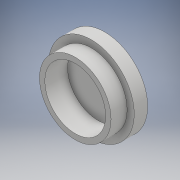
# Autodesk Inventor part: CapForPh
Saved by Autodesk Inventor 2019 (Build 230136000, 136)
## iProperties
Created: 2017-07-24
Part Number: CapForPh
Material: Generic
Document SubType Name: Modeling
Designer: steele
Density: 1 g/cm^3
Appearance: Default
Author: steele
Autodesk Inventor part; units mm, degrees
ref_plane "YZ Plane" through (0, 0, 0) normal (1, 0, 0) x (0, 1, 0)
ref_plane "XZ Plane" through (0, 0, 0) normal (0, 1, 0) x (-1, 0, 0)
ref_plane "XY Plane" through (0, 0, 0) normal (0, 0, 1) x (1, 0, 0)
sketch "Sketch2" plane through (0, 0, 0) normal (0, 0, 1) x (1, 0, 0)
  line L0 (0, 0) -> (0, 11) construction
  line L1 (0, 11) -> (-16, 11)
  line L2 (-16, 11) -> (-16, 6)
  line L3 (-16, 6) -> (-13.35, 6)
  line L4 (-13.35, 6) -> (-13.35, 0)
  line L5 (-13.35, 0) -> (-11.35, 0)
  line L6 (0, 0) -> (-13.35, 0) construction
  line L7 (-11.35, 0) -> (-11.35, 6)
  line L8 (0, 11) -> (0, 8.5)
  line L9 (-11.35, 8.5) -> (-11.35, 6)
  line L10 (-11.35, 8.5) -> (0, 8.5)
  dimension "d4" = 16
  dimension "d5" = 5
  dimension "d6" = 6
  dimension "d8" = 13.35
  dimension "d16" = 11.35
  dimension "d17" = 2
  constraints: 22 end point, 5 perpendicular, 3 vertical, 2 point on line, 1 collinear, 1 horizontal, 1 parallel
  measures "d4" distance of L0.end L1.end
  measures "d5" distance of L1.end L2.end
  measures "d6" distance of L3.end L4.end
  measures "d8" distance between parallel lines of L0 L4
  measures "d16" distance between parallel lines of L7 L0
  measures "d17" distance between parallel lines of L7 L4
revolve "Revolution1" add sketch "Sketch2" angle 360 about axis through (0, 0, 0) along (0, 1, 0)
sketch "Sketch4" plane through (0, 11, 0) normal (0, 1, 0) x (1, 0, 0)
  circle A0 centre (0, 0) radius 16 construction
  line L0 (-16, 0) -> (16, 0) construction
  spline S0 degree 2 poles (-9.9681, -0.6371) (-9.9681, -1.7395) (-11.0853, -3.089) (-11.9059, -3.089) knots 0 0 0 1 2 2 2
  spline S1 degree 2 poles (-11.9059, -3.089) (-12.247, -3.089) (-12.7561, -2.9357) (-13.0428, -2.7677) knots 0 0 0 1 2 2 2
  line L1 (-13.0428, -2.7677) -> (-13.0428, -4.6857)
  line L2 (-13.0428, -4.6857) -> (-14.4764, -4.6857)
  line L3 (-14.4764, -4.6857) -> (-14.4764, 1.6022)
  line L4 (-14.4764, 1.6022) -> (-13.0428, 1.6022)
  line L5 (-13.0428, 1.6022) -> (-13.0428, 1.1177)
  spline S2 degree 2 poles (-13.0428, 1.1177) (-12.7265, 1.3896) (-12.0739, 1.7258) (-11.6439, 1.7258) knots 0 0 0 1 2 2 2
  spline S3 degree 2 poles (-11.6439, 1.7258) (-10.8431, 1.7258) (-9.9681, 0.4553) (-9.9681, -0.6371) knots 0 0 0 1 2 2 2
  spline S4 degree 2 poles (-11.4363, -0.6668) (-11.4363, 0.0055) (-11.8515, 0.6086) (-12.2865, 0.6086) knots 0 0 0 1 2 2 2
  spline S5 degree 2 poles (-12.2865, 0.6086) (-12.4793, 0.6086) (-12.8599, 0.485) (-13.0428, 0.3614) knots 0 0 0 1 2 2 2
  line L6 (-13.0428, 0.3614) -> (-13.0428, -1.9471)
  spline S6 degree 2 poles (-13.0428, -1.9471) (-12.9291, -1.9965) (-12.6523, -2.0361) (-12.4645, -2.0361) knots 0 0 0 1 2 2 2
  spline S7 degree 2 poles (-12.4645, -2.0361) (-11.9454, -2.0361) (-11.4363, -1.3539) (-11.4363, -0.6668) knots 0 0 0 1 2 2 2
  line L7 (-3.967, -3) -> (-5.4994, -3)
  line L8 (-5.4994, -3) -> (-5.4994, -0.296)
  line L9 (-5.4994, -0.296) -> (-7.5805, -0.296)
  line L10 (-7.5805, -0.296) -> (-7.5805, -3)
  line L11 (-7.5805, -3) -> (-9.1129, -3)
  line L12 (-9.1129, -3) -> (-9.1129, 3.1)
  line L13 (-9.1129, 3.1) -> (-7.5805, 3.1)
  line L14 (-7.5805, 3.1) -> (-7.5805, 0.8656)
  line L15 (-7.5805, 0.8656) -> (-5.4994, 0.8656)
  line L16 (-5.4994, 0.8656) -> (-5.4994, 3.1)
  line L17 (-5.4994, 3.1) -> (-3.967, 3.1)
  line L18 (-3.967, 3.1) -> (-3.967, -3)
  spline S8 degree 2 poles (2.3851, -3.1186) (1.0109, -3.1186) (-0.6006, -1.4577) (-0.6006, 0.0451) knots 0 0 0 1 2 2 2
  spline S9 degree 2 poles (-0.6006, 0.0451) (-0.6006, 1.4934) (1.0158, 3.2186) (2.3901, 3.2186) knots 0 0 0 1 2 2 2
  spline S10 degree 2 poles (2.3901, 3.2186) (2.7509, 3.2186) (3.3342, 3.1346) (3.6012, 3.0654) knots 0 0 0 1 2 2 2
  spline S11 degree 2 poles (3.6012, 3.0654) (3.8088, 3.0011) (4.2982, 2.7886) (4.4514, 2.7095) knots 0 0 0 1 2 2 2
  line L19 (4.4514, 2.7095) -> (4.4514, 1.2562)
  line L20 (4.4514, 1.2562) -> (4.2982, 1.2562)
  spline S12 degree 2 poles (4.2982, 1.2562) (4.1845, 1.355) (3.8483, 1.6318) (3.6358, 1.7604) knots 0 0 0 1 2 2 2
  spline S13 degree 2 poles (3.6358, 1.7604) (3.4232, 1.8938) (2.9141, 2.0767) (2.6323, 2.0767) knots 0 0 0 1 2 2 2
  spline S14 degree 2 poles (2.6323, 2.0767) (2.3011, 2.0767) (1.7524, 1.8691) (1.5003, 1.6071) knots 0 0 0 1 2 2 2
  spline S15 degree 2 poles (1.5003, 1.6071) (1.2729, 1.3748) (0.9812, 0.5789) (0.9812, 0.0401) knots 0 0 0 1 2 2 2
  spline S16 degree 2 poles (0.9812, 0.0401) (0.9812, -0.5284) (1.2828, -1.3045) (1.5299, -1.5417) knots 0 0 0 1 2 2 2
  spline S17 degree 2 poles (1.5299, -1.5417) (1.7672, -1.7741) (2.3505, -1.9767) (2.6422, -1.9767) knots 0 0 0 1 2 2 2
  spline S18 degree 2 poles (2.6422, -1.9767) (2.9437, -1.9767) (3.4924, -1.7741) (3.6803, -1.6505) knots 0 0 0 1 2 2 2
  spline S19 degree 2 poles (3.6803, -1.6505) (3.8879, -1.5269) (4.1993, -1.2649) (4.313, -1.1611) knots 0 0 0 1 2 2 2
  line L21 (4.313, -1.1611) -> (4.4514, -1.1611)
  line L22 (4.4514, -1.1611) -> (4.4514, -2.5947)
  spline S20 degree 2 poles (4.4514, -2.5947) (4.2833, -2.6737) (3.8434, -2.8715) (3.6061, -2.9407) knots 0 0 0 1 2 2 2
  spline S21 degree 2 poles (3.6061, -2.9407) (3.3194, -3.0297) (2.8201, -3.1186) (2.3851, -3.1186) knots 0 0 0 1 2 2 2
  spline S22 degree 2 poles (7.8079, -2.5106) (7.6596, -2.6342) (7.4273, -2.8319) (7.2295, -2.9308) knots 0 0 0 1 2 2 2
  spline S23 degree 2 poles (7.2295, -2.9308) (7.0367, -3.0247) (6.6709, -3.1236) (6.3447, -3.1236) knots 0 0 0 1 2 2 2
  spline S24 degree 2 poles (6.3447, -3.1236) (5.7317, -3.1236) (4.926, -2.303) (4.926, -1.6801) knots 0 0 0 1 2 2 2
  spline S25 degree 2 poles (4.926, -1.6801) (4.926, -1.171) (5.3363, -0.5382) (5.7218, -0.3553) knots 0 0 0 1 2 2 2
  spline S26 degree 2 poles (5.7218, -0.3553) (6.1124, -0.1675) (7.1949, -0.0192) (7.8178, 0.0203) knots 0 0 0 1 2 2 2
  line L23 (7.8178, 0.0203) -> (7.8178, 0.0451)
  spline S27 degree 2 poles (7.8178, 0.0451) (7.8178, 0.4257) (7.2543, 0.7173) (6.6907, 0.7173) knots 0 0 0 1 2 2 2
  spline S28 degree 2 poles (6.6907, 0.7173) (6.4386, 0.7173) (5.7564, 0.5344) (5.4351, 0.3911) knots 0 0 0 1 2 2 2
  line L24 (5.4351, 0.3911) -> (5.3115, 0.3911)
  line L25 (5.3115, 0.3911) -> (5.3115, 1.5033)
  spline S29 degree 2 poles (5.3115, 1.5033) (5.5241, 1.5626) (6.4732, 1.7307) (6.9577, 1.7307) knots 0 0 0 1 2 2 2
  spline S30 degree 2 poles (6.9577, 1.7307) (8.144, 1.7307) (9.2316, 0.9398) (9.2316, 0.1291) knots 0 0 0 1 2 2 2
  line L26 (9.2316, 0.1291) -> (9.2316, -3)
  line L27 (9.2316, -3) -> (7.8079, -3)
  line L28 (7.8079, -3) -> (7.8079, -2.5106)
  line L29 (7.8079, -1.7988) -> (7.8079, -0.8447)
  spline S31 degree 2 poles (7.8079, -0.8447) (7.4421, -0.8793) (6.9923, -0.9337) (6.7748, -1.0128) knots 0 0 0 1 2 2 2
  spline S32 degree 2 poles (6.7748, -1.0128) (6.582, -1.0771) (6.3744, -1.344) (6.3744, -1.5615) knots 0 0 0 1 2 2 2
  spline S33 degree 2 poles (6.3744, -1.5615) (6.3744, -1.8828) (6.7253, -2.125) (7.0664, -2.125) knots 0 0 0 1 2 2 2
  spline S34 degree 2 poles (7.0664, -2.125) (7.2543, -2.125) (7.6497, -1.952) (7.8079, -1.7988) knots 0 0 0 1 2 2 2
  spline S35 degree 2 poles (14.8026, -0.6371) (14.8026, -1.7395) (13.6855, -3.089) (12.8649, -3.089) knots 0 0 0 1 2 2 2
  spline S36 degree 2 poles (12.8649, -3.089) (12.5238, -3.089) (12.0146, -2.9357) (11.7279, -2.7677) knots 0 0 0 1 2 2 2
  line L30 (11.7279, -2.7677) -> (11.7279, -4.6857)
  line L31 (11.7279, -4.6857) -> (10.2944, -4.6857)
  line L32 (10.2944, -4.6857) -> (10.2944, 1.6022)
  line L33 (10.2944, 1.6022) -> (11.7279, 1.6022)
  line L34 (11.7279, 1.6022) -> (11.7279, 1.1177)
  spline S37 degree 2 poles (11.7279, 1.1177) (12.0443, 1.3896) (12.6968, 1.7258) (13.1269, 1.7258) knots 0 0 0 1 2 2 2
  spline S38 degree 2 poles (13.1269, 1.7258) (13.9277, 1.7258) (14.8026, 0.4553) (14.8026, -0.6371) knots 0 0 0 1 2 2 2
  spline S39 degree 2 poles (13.3345, -0.6668) (13.3345, 0.0055) (12.9192, 0.6086) (12.4842, 0.6086) knots 0 0 0 1 2 2 2
  spline S40 degree 2 poles (12.4842, 0.6086) (12.2914, 0.6086) (11.9108, 0.485) (11.7279, 0.3614) knots 0 0 0 1 2 2 2
  line L35 (11.7279, 0.3614) -> (11.7279, -1.9471)
  spline S41 degree 2 poles (11.7279, -1.9471) (11.8416, -1.9965) (12.1184, -2.0361) (12.3063, -2.0361) knots 0 0 0 1 2 2 2
  spline S42 degree 2 poles (12.3063, -2.0361) (12.8253, -2.0361) (13.3345, -1.3539) (13.3345, -0.6668) knots 0 0 0 1 2 2 2
  point P0 (0, 0)
  constraints: 2 end point, 2 horizontal, 2 point on circle
extrude "Extrusion2" cut sketch "Sketch4" against normal blind 2
body "Solid1"
